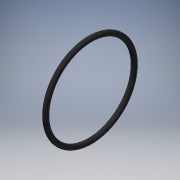
# Autodesk Inventor part: 9396K153 Silicone O-Ring
Saved by Autodesk Inventor 2019.4 (Build 234330000, 330)
## iProperties
Created: 2012-06-04
Part Number: 9396K153 Silicone O-Ring
Material: Rubber, Silicone
Document SubType Name: Modeling
Designer: ding42
Mass: 0.980917 g
Surface Area: 12.0333 cm^2
Volume: 0.784734 cm^3
Density: 1.25 g/cm^3
Description: Dash Number 132
Appearance: Rubber - Black
Author: ding42
Autodesk Inventor part; units mm, degrees
ref_plane "YZ Plane" through (0, 0, 0) normal (1, 0, 0) x (0, 1, 0)
ref_plane "XZ Plane" through (0, 0, 0) normal (0, 1, 0) x (-1, 0, 0)
ref_plane "XY Plane" through (0, 0, 0) normal (0, 0, 1) x (1, 0, 0)
sketch "Sketch1" plane through (0, 0, 0) normal (0, 0, 1) x (1, 0, 0)
  circle A0 centre (0, 0) radius 1.3081
  dimension "d0" = 2.6162
  constraints: 1 centre point, 1 coincident
  measures "d0" diameter of A0
sketch "Sketch2" plane through (0, 0, 0) normal (1, 0, 0) x (0, 1, 0)
  circle A0 centre (23.2333, -2.4338) radius 22.0599
  circle A1 centre (23.2333, -2.4338) radius 24.6761 construction
  line L0 (1.3081, 0) -> (-1.3081, 0) projected
  point P0 (0, 0)
  dimension "d1" = 44.1198
  dimension "d2" = 49.3522
  constraints: 1 centre point, 1 coincident, 3 other
  measures "d2" diameter of A1
sweep "Sweep1" add profiles "Sketch1" path "Sketch2" path curves A0
body "Solid1"
